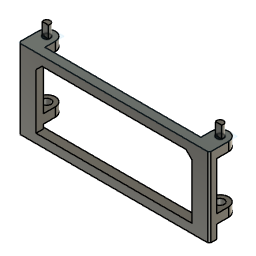
Raspberry PI Bracket (Autodesk Fusion 360 design; units mm, degrees)
Autodesk Fusion 360 part; units mm, degrees
sketch "Sketch1" plane through (0, 0, 0) normal (0, 1, 0) x (1, 0, 0)
  line L0 (0, 0) -> (63.8, 0)
  line L1 (63.8, 0) -> (63.8, -22)
  line L2 (63.8, -22) -> (0, -22)
  line L3 (0, -22) -> (0, 0)
  line L4 (0, 0) -> (0, 1.4)
  line L5 (0, 1.4) -> (0, 4.4)
  line L6 (0, 4.4) -> (63.8, 4.4)
  line L7 (0, 1.4) -> (63.8, 1.4)
  line L8 (63.8, 1.4) -> (63.8, 0)
  line L9 (63.8, 4.4) -> (63.8, 1.4)
  line L10 (0, -19) -> (63.8, -19)
  line L11 (5.8, 4.4) -> (5.8, -22)
  line L12 (58, 4.4) -> (58, -22)
  line L13 (0, -3) -> (63.8, -3)
  dimension "d1" = 63.8
  dimension "d2" = 22
  dimension "d3" = 1.4
  dimension "d4" = 3
  dimension "d5" = 3
  dimension "d6" = 5.8
  dimension "d7" = 5.8
  dimension "d28" = 3
  constraint horizontal L0
  constraint vertical L1
  constraint horizontal L2
  constraint vertical L3
  constraint coincident L0.start L3.end
  constraint vertical L4
  constraint parallel L4 L5
  constraint perpendicular L5 L6
  constraint perpendicular L4 L7
  constraint perpendicular L7 L8
  constraint perpendicular L6 L9
  constraint coincident L3 L10.start
  constraint coincident L1 L10.end
  constraint perpendicular L1 L10
  constraint coincident L6 L11.start
  constraint coincident L2 L11.end
  constraint perpendicular L2 L11
  constraint coincident L6 L12.start
  constraint coincident L2 L12.end
  constraint perpendicular L2 L12
  constraint coincident L3 L13.start
  constraint coincident L1 L13.end
  constraint perpendicular L1 L13
  measures "d1" distance of L1.end L2.end
  measures "d2" distance of L0.start L2.end
  measures "d3" distance of L0 L7
  measures "d4" distance of L6 L7
  measures "d5" distance of L2 L10
  measures "d6" distance of L1 L12
  measures "d7" distance of L3 L11
  measures "d28" distance of L0 L13
extrude "Extrude1" add sketch "Sketch1" against normal blind 3 contours L0 L4 L7 L11 | L0 L3 L11 L13 | L3 L10 L11 L13 | L5 L6 L7 L11 | L0 L7 L8 L12 | L0 L1 L12 L13 | L6 L7 L11 L12 | L2 L3 L10 L11 | L6 L7 L9 L12 | L1 L10 L12 L13 | L2 L10 L11 L12 | L1 L2 L10 L12 makes body 1
extrude "Extrude2" add sketch "Sketch1" along normal blind 6.4 contours L0 L3 L11 L13 | L0 L1 L12 L13 | L2 L3 L10 L11 | L1 L2 L10 L12 bodies 1
move_face "OffsetFaces1" [suppressed]
hole "Hole1" at (2.9, 3.5, 0) direction (0, 0, 1) diameter 2.9 depth 6 tip angle 118 bodies 1
hole "Hole2" at (60.9, 3.5, 0) direction (0, 0, 1) diameter 2.9 depth 9 tip angle 118 bodies 1
sketch "Sketch2" plane through (0, 0, 22) normal (0, 0, 1) x (-1, 0, 0)
  line L0 (-58, 0) -> (-5.8, 0)
  line L1 (-5.8, 0) -> (-5.8, -6.4)
  line L2 (-5.8, -6.4) -> (0, -6.4)
  line L3 (0, -6.4) -> (0, 3)
  line L4 (0, 3) -> (-63.8, 3)
  line L5 (-63.8, 3) -> (-63.8, -6.4)
  line L6 (-63.8, -6.4) -> (-58, -6.4)
  line L7 (-58, -6.4) -> (-58, 0)
  circle A0 centre (-2.9, -3.5) radius 1.15
  circle A1 centre (-60.9, -3.5) radius 1.15
  line L8 (-61.9356, -3) -> (-59.8644, -3)
  line L9 (-3.9356, -3) -> (-1.8644, -3)
  dimension "d34" = 2.9
  dimension "d35" = 2.9
  dimension "d36" = 2.9
  dimension "d37" = 2.9
  dimension "d38" = 2.3
  dimension "d41" = 0.5
  dimension "d42" = 0.5
  constraint equal A0 A1
  constraint coincident A1 L8.start
  constraint coincident A1 L8.end
  constraint horizontal L8
  constraint coincident A0 L9.start
  constraint coincident A0 L9.end
  constraint perpendicular L7 L9
  measures "d34" distance of L6 A1.centre
  measures "d35" distance of L5 A1.centre
  measures "d36" distance of L2 A0.centre
  measures "d37" distance of L3 A0.centre
  measures "d38" diameter of A0
  measures "d41" distance of A1.centre L8
  measures "d42" distance of A0.centre L9
extrude "Extrude3" add sketch "Sketch2" along normal mid plane 8 separate body contours A0 L9 | A0 L9 | A1 L8 | A1 L8 makes body 2 at (2.2289, 4.4339, 24.6667) makes body 3 at (61.7035, 4.3227, 24.6667)
combine "Combine1" operation cut target body 1 tool bodies 3 2 keep tools
extrude "Extrude4" cut sketch "Sketch2" along normal mid plane 8 contours A0 L9 | A1 L8 picked at (-2.6192, -2.9057) picked at (-60.9208, -2.6987) bodies 2 3
fillet "Fillet2" radius 2.9 8 edges at (0, 6.4, 1.5) (0, 6.4, 20.5) (5.8, 6.4, 1.5) (58, 6.4, 1.5) (63.8, 6.4, 20.5) (63.8, 6.4, 1.5) (58, 6.4, 20.5) (5.8, 6.4, 20.5) on bodies 1
chamfer "Chamfer3" distance 2 angle 45 2 edges at (5.8, -1.5, 19) (58, -1.5, 19) on bodies 1
chamfer "Chamfer4" distance 0.5 angle 45 9 edges at (0, -3, 8.8) (63.8, -3, 8.8) (0, 0, -2.2) (0, 0, 11) (5.8, 0, -0.7) (5.8, 0, 11) (58, 0, -0.7) (63.8, 0, 11) (63.8, 0, -2.2) on bodies 1
chamfer "Chamfer7" distance 1 angle 45 2 edges at (60.9, 4.65, 18) (2.9, 4.65, 18) on bodies 2 3
equation "d1 = 58 mm + 5.8 mm"
equation "d10 = 3.5 mm + ( 5.8 / 2 ) * 1 mm"
equation "d15 = ( 5.8 / 2 ) * 1 mm"
equation "d16 = ( 5.8 / 2 ) * 1 mm"
equation "d20 = ( 5.8 / 2 ) * 1 mm"
equation "d21 = ( 5.8 / 2 ) * 1 mm"
equation "d33 = ( 5.8 / 2 ) * 1 mm"
equation "d34 = ( 5.8 / 2 ) * 1 mm"
equation "d35 = ( 5.8 / 2 ) * 1 mm"
equation "d36 = ( 5.8 / 2 ) * 1 mm"
equation "d37 = ( 5.8 / 2 ) * 1 mm"
